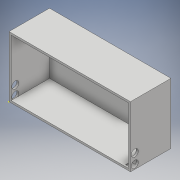
# Autodesk Inventor part: Pieza2
Saved by Autodesk Inventor 2017 (Build 210142000, 142)
## iProperties
Part Number: Pieza2
Material: Genérico
Document SubType Name: Modeling
Designer: diego
Density: 1 g/cm^3
Appearance: Valor por defecto
Author: diego
Autodesk Inventor part; units mm, degrees
ref_plane "YZ Plane" through (0, 0, 0) normal (1, 0, 0) x (0, 1, 0)
ref_plane "XZ Plane" through (0, 0, 0) normal (0, 1, 0) x (-1, 0, 0)
ref_plane "XY Plane" through (0, 0, 0) normal (0, 0, 1) x (1, 0, 0)
sketch "Boceto1" plane through (0, 0, 0) normal (0, 0, 1) x (1, 0, 0)
  point P0 (0, 0)
sketch "Boceto2" plane through (0, 0, 0) normal (0, 0, 1) x (1, 0, 0)
  line L0 (0, 0) -> (0, 200)
  line L1 (0, 200) -> (600, 200)
  line L2 (600, 200) -> (600, 0)
  line L3 (600, 0) -> (0, 0)
  dimension "d0" = 200
  dimension "d1" = 600
  dimension "d2" = 200
  dimension "d3" = 600
  constraints: 8 end point, 2 perpendicular, 1 vertical
  measures "d0" distance of L0.start L0.end
  measures "d1" distance of L0.end L1.end
  measures "d2" distance of L1.end L2.end
  measures "d3" distance of L2.end L0.start
extrude "Extrusión1" add sketch "Boceto2" along normal blind 300
shell "Vaciado1" thickness 10 removed faces 1 at (400, 0, 100)
sketch "Boceto3" plane through (0, 200, 0) normal (0, 1, 0) x (1, 0, 0)
  point P0 (0, 0)
sketch "Boceto4" plane through (0, 200, 0) normal (0, 1, 0) x (1, 0, 0)
  point P0 (0, 0)
sketch "Boceto5" plane through (0, 200, 0) normal (0, 1, 0) x (1, 0, 0)
  point P0 (0, 0)
sketch "Boceto6" plane through (0, 200, 0) normal (0, 1, 0) x (1, 0, 0)
  circle A0 centre (300, -150) radius 15
  point P0 (0, 0)
  dimension "d9" = 30
  constraints: 1 centre point
  measures "d9" diameter of A0
extrude "Extrusión2" cut sketch "Boceto6" against normal blind 33.25
sketch "Boceto7" plane through (0, 200, 0) normal (0, 1, 0) x (1, 0, 0)
  point P0 (0, 0)
sketch "Boceto8" plane through (600, 0, 0) normal (1, 0, 0) x (0, 0, -1)
  circle A0 centre (-22.0681, 21.036) radius 17.5
  circle A1 centre (-69.9749, 21.036) radius 17.5
  point P0 (0, 0)
  dimension "d12" = 35
  dimension "d13" = 35
  constraints: 2 centre point
  measures "d12" diameter of A0
  measures "d13" diameter of A1
extrude "Extrusión3" cut sketch "Boceto8" against normal blind 33.25
sketch "Boceto9" plane through (0, 0, 0) normal (-1, 0, 0) x (0, 0, 1)
  arc A0 (10, 8.3628) -> (10, 33.7092) centre (22.0681, 21.036) ccw projected
  circle A1 centre (22.0681, 21.036) radius 17.5
  circle A2 centre (66.1324, 21.036) radius 17.5
  point P0 (0, 0)
  dimension "d16" = 35
  dimension "d17" = 35
  constraints: 2 centre point, 1 coincident
  measures "d16" diameter of A1
  measures "d17" diameter of A2
extrude "Extrusión4" cut sketch "Boceto9" against normal blind 10
